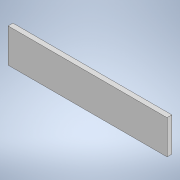
# Autodesk Inventor part: frontOfHouseUnder Deck
Saved by Autodesk Inventor 2020.1 (Build 241239000, 239)
## iProperties
Created: 2019-08-11
Part Number: frontOfHouseUnder Deck
Material: Generic
Document SubType Name: Modeling
Designer: steele
Density: 1 g/cm^3
Appearance: Default
Author: steele
Autodesk Inventor part; units mm, degrees
ref_plane "YZ Plane" through (0, 0, 0) normal (1, 0, 0) x (0, 1, 0)
ref_plane "XZ Plane" through (0, 0, 0) normal (0, 1, 0) x (-1, 0, 0)
ref_plane "XY Plane" through (0, 0, 0) normal (0, 0, 1) x (1, 0, 0)
sketch "Sketch1" plane through (0, 0, 0) normal (0, 0, 1) x (1, 0, 0)
  line L0 (0, 0) -> (-4978.4, 0)
  line L1 (-4978.4, 0) -> (-4978.4, 2133.6)
  line L2 (-4978.4, 2133.6) -> (0, 2133.6)
  line L3 (0, 2133.6) -> (0, 0)
  line L4 (0, 0) -> (5003.8, 0)
  line L5 (5003.8, 0) -> (5003.8, 2133.6)
  line L6 (5003.8, 2133.6) -> (0, 2133.6)
  line L7 (0, 2133.6) -> (0, 0)
  dimension "d0" = 4978.4
  dimension "d1" = 2133.6
  dimension "d2" = 5003.8
  dimension "d3" = 2133.6
  constraints: 16 end point, 4 parallel, 2 horizontal, 2 perpendicular
  measures "d0" distance of L1.end L2.end
  measures "d1" distance of L0.end L1.end
  measures "d2" distance of L6.end L5.end
  measures "d3" distance of L5.end L4.end
extrude "Extrusion1" add sketch "Sketch1" against normal blind 304.8
body "Solid1"
